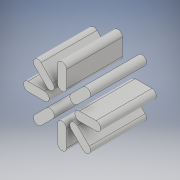
# Autodesk Inventor part: location hole
Saved by Autodesk Inventor 2019 (Build 230136000, 136)
## iProperties
Created: 2018-10-02
Part Number: location hole
Material: Generic
Document SubType Name: Modeling
Designer: HIVE
Density: 1 g/cm^3
Appearance: Default
Author: HIVE
Autodesk Inventor part; units mm, degrees
ref_plane "YZ Plane" through (0, 0, 0) normal (1, 0, 0) x (0, 1, 0)
ref_plane "XZ Plane" through (0, 0, 0) normal (0, 1, 0) x (-1, 0, 0)
ref_plane "XY Plane" through (0, 0, 0) normal (0, 0, 1) x (1, 0, 0)
sketch "Sketch1" plane through (0, 0, 0) normal (0, 0, 1) x (1, 0, 0)
  line L0 (0, 30.4699) -> (0, 15.4699) construction
  line L1 (4, 30.4699) -> (4, 15.4699)
  line L2 (-4, 15.4699) -> (-4, 30.4699)
  arc A0 (4, 30.4699) -> (-4, 30.4699) centre (0, 30.4699) ccw
  arc A1 (-4, 15.4699) -> (4, 15.4699) centre (0, 15.4699) ccw
  circle A2 centre (0, 0) radius 22.9699 construction
  arc A3 (-18.717, 24.3739) -> (-24.3739, 18.717) centre (-21.5455, 21.5455) ccw
  line L3 (-18.717, 24.3739) -> (-8.1104, 13.7673)
  arc A4 (-13.7673, 8.1104) -> (-8.1104, 13.7673) centre (-10.9389, 10.9389) ccw
  line L4 (-13.7673, 8.1104) -> (-24.3739, 18.717)
  circle A5 centre (0, 0) radius 22.9699 construction
  arc A6 (-30.4699, 4) -> (-30.4699, -4) centre (-30.4699, 0) ccw
  line L5 (-30.4699, 4) -> (-15.4699, 4)
  arc A7 (-15.4699, -4) -> (-15.4699, 4) centre (-15.4699, 0) ccw
  line L6 (-15.4699, -4) -> (-30.4699, -4)
  circle A8 centre (0, 0) radius 22.9699 construction
  arc A9 (-24.3739, -18.717) -> (-18.717, -24.3739) centre (-21.5455, -21.5455) ccw
  line L7 (-24.3739, -18.717) -> (-13.7673, -8.1104)
  arc A10 (-8.1104, -13.7673) -> (-13.7673, -8.1104) centre (-10.9389, -10.9389) ccw
  line L8 (-8.1104, -13.7673) -> (-18.717, -24.3739)
  circle A11 centre (0, 0) radius 22.9699 construction
  arc A12 (-4, -30.4699) -> (4, -30.4699) centre (0, -30.4699) ccw
  line L9 (-4, -30.4699) -> (-4, -15.4699)
  arc A13 (4, -15.4699) -> (-4, -15.4699) centre (0, -15.4699) ccw
  line L10 (4, -15.4699) -> (4, -30.4699)
  circle A14 centre (0, 0) radius 22.9699 construction
  arc A15 (18.717, -24.3739) -> (24.3739, -18.717) centre (21.5455, -21.5455) ccw
  line L11 (18.717, -24.3739) -> (8.1104, -13.7673)
  arc A16 (13.7673, -8.1104) -> (8.1104, -13.7673) centre (10.9389, -10.9389) ccw
  line L12 (13.7673, -8.1104) -> (24.3739, -18.717)
  circle A17 centre (0, 0) radius 22.9699 construction
  arc A18 (30.4699, -4) -> (30.4699, 4) centre (30.4699, 0) ccw
  line L13 (30.4699, -4) -> (15.4699, -4)
  arc A19 (15.4699, 4) -> (15.4699, -4) centre (15.4699, 0) ccw
  line L14 (15.4699, 4) -> (30.4699, 4)
  circle A20 centre (0, 0) radius 22.9699 construction
  arc A21 (24.3739, 18.717) -> (18.717, 24.3739) centre (21.5455, 21.5455) ccw
  line L15 (24.3739, 18.717) -> (13.7673, 8.1104)
  arc A22 (8.1104, 13.7673) -> (13.7673, 8.1104) centre (10.9389, 10.9389) ccw
  line L16 (8.1104, 13.7673) -> (18.717, 24.3739)
  circle A23 centre (0, 0) radius 22.9699 construction
  point P0 (0, 22.9699)
  point P1 (-16.2422, 16.2422)
  point P2 (-22.9699, 0)
  point P3 (-16.2422, -16.2422)
  point P4 (0, -22.9699)
  point P5 (16.2422, -16.2422)
  point P6 (22.9699, 0)
  point P7 (16.2422, 16.2422)
  dimension "d0" = 4
  dimension "d1" = 15
  dimension "d4" = 360
  constraints: 36 end point, 32 point on circle, 16 centre point, 4 tangent, 3 coincident, 2 horizontal alignment, 2 vertical alignment, 1 midpoint, 1 parallel, 1 vertical, 123 other
  measures "d0" radius of A1
  measures "d1" distance of L0.start L0.end
extrude "Extrusion1" add sketch "Sketch1" along normal blind 50
body "Solid1"
